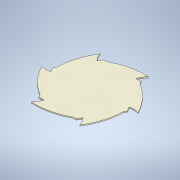
# Autodesk Inventor part: Hex_Nexus
Saved by Autodesk Inventor 2021 (Build 250183000, 183)
## iProperties
Created: 2023-03-16
Part Number: Hex_Nexus
Material: Paper
Document SubType Name: Modeling
Designer: Bradley
Density: 0.93 g/cm^3
Appearance: Cardboard - Chipboard
Author: Bradley
Autodesk Inventor part; units mm, degrees
ref_plane "YZ Plane" through (0, 0, 0) normal (1, 0, 0) x (0, 1, 0)
ref_plane "XZ Plane" through (0, 0, 0) normal (0, 1, 0) x (-1, 0, 0)
ref_plane "XY Plane" through (0, 0, 0) normal (0, 0, 1) x (1, 0, 0)
sketch "Sketch1" plane through (0, 0, 0) normal (0, 1, 0) x (-1, 0, 0)
  line L0 (-29.1562, -50.5) -> (-58.3124, 0)
  line L1 (-58.3124, 0) -> (-29.1562, 50.5)
  line L2 (-29.1562, 50.5) -> (29.1562, 50.5)
  line L3 (29.1562, 50.5) -> (58.3124, 0)
  line L4 (58.3124, 0) -> (29.1562, -50.5)
  line L5 (29.1562, -50.5) -> (-29.1562, -50.5)
  arc A0 (-28.4819, -62.5624) -> (-21.4664, -50.5) centre (-45.317, -44.6997) ccw
  arc A1 (-28.4819, -62.5624) -> (24.1797, -50.5) centre (-23.0158, 34.5591) ccw
  line L6 (24.1797, -50.5) -> (-21.4664, -50.5)
  arc A2 (39.9397, -55.9473) -> (33.0011, -43.8404) centre (16.0526, -61.5955) ccw
  arc A3 (39.9397, -55.9473) -> (55.8241, -4.3097) centre (-41.437, -2.6527) ccw
  line L7 (55.8241, -4.3097) -> (33.0011, -43.8404)
  arc A4 (68.4216, 6.6151) -> (54.4675, 6.6596) centre (61.3696, -16.8958) ccw
  arc A5 (68.4216, 6.6151) -> (31.6444, 46.1903) centre (-18.4211, -37.2118) ccw
  line L8 (31.6444, 46.1903) -> (54.4675, 6.6596)
  arc A6 (28.4819, 62.5624) -> (21.4664, 50.5) centre (45.317, 44.6997) ccw
  arc A7 (28.4819, 62.5624) -> (-24.1797, 50.5) centre (23.0158, -34.5591) ccw
  line L9 (-24.1797, 50.5) -> (21.4664, 50.5)
  arc A8 (-39.9397, 55.9473) -> (-33.0011, 43.8404) centre (-16.0526, 61.5955) ccw
  arc A9 (-39.9397, 55.9473) -> (-55.8241, 4.3097) centre (41.437, 2.6527) ccw
  line L10 (-55.8241, 4.3097) -> (-33.0011, 43.8404)
  arc A10 (-68.4216, -6.6151) -> (-54.4675, -6.6596) centre (-61.3696, 16.8958) ccw
  arc A11 (-68.4216, -6.6151) -> (-31.6444, -46.1903) centre (18.4211, 37.2118) ccw
  line L11 (-31.6444, -46.1903) -> (-54.4675, -6.6596)
  point P0 (0, 0)
  point P1 (0, 0)
  point P2 (31.6444, 46.1903)
  point P3 (54.4675, 6.6596)
  point P4 (-24.1797, 50.5)
  point P5 (21.4664, 50.5)
  point P6 (-55.8241, 4.3097)
  point P7 (-31.6444, -46.1903)
  point P8 (-54.4675, -6.6596)
  point P9 (55.8241, -4.3097)
  point P10 (33.0011, -43.8404)
  dimension "d0" = 101
  dimension "d19" = 360
  dimension "d21" = 24.5458
  dimension "d22" = 97.2752
  dimension "d23" = 4.9765
  dimension "d24" = 7.6898
  constraints: 24 end point, 24 point on circle, 12 centre point, 2 point on line, 1 coincident, 1 collinear, 1 horizontal, 64 other
  measures "d0" distance between parallel lines of L2 L5
  measures "d21" radius of A0
  measures "d22" radius of A1
  measures "d23" distance of L6.start L4.end
  measures "d24" distance of L6.end L0.start
extrude "Extrusion1" add sketch "Sketch1" along normal blind 1.7
body "Solid1"
